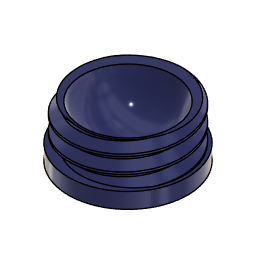
joint attachments v8 (Autodesk Fusion 360 archive; units mm, degrees)
design "thread"
Autodesk Fusion 360 part; units mm, degrees
sketch "Ball" plane through (0, 0, 0) normal (1, 0, 0) x (0, 1, 0)
  circle A0 centre (0, 0) radius 9 construction
  line L0 (0, 0) -> (0, 4.9749) construction
  line L1 (0, 4.9749) -> (-7.5, 4.9749) construction
  line L2 (-7.5, 4.9749) -> (-7.5, 0) construction
  line L3 (-7.5, 0) -> (-9, 0) construction
  line L4 (0, 0) -> (0, -2) construction
  line L5 (0, -2) -> (-8.775, -2) construction
  line L6 (0, -2) -> (0, -9) construction
  dimension "d58" = 18
  dimension "d109" = 2
  dimension "d110" = 1.5
  constraint coincident A0.centre L0.start
  constraint vertical L0
  constraint coincident A0 L1.end
  constraint perpendicular L0 L1
  constraint perpendicular L1 L2
  constraint coincident A0 L3.end
  constraint horizontal L3
  constraint coincident A0.centre L3
  constraint vertical L4
  constraint coincident A0 L5.end
  constraint perpendicular L4 L5
  constraint coincident A0 L6.end
  constraint perpendicular L5 L6
  measures "d58" diameter of A0
  measures "d109" distance of A0.centre L4.end
  measures "d110" distance of L2.end L3.end
sketch "Sketch1" plane through (0, 0, 0) normal (1, 0, 0) x (0, 1, 0) in component "Socket"
  circle A0 centre (0, 0) radius 9
  line L0 (0, -9) -> (-11.5, -9)
  line L1 (0, -12) -> (-11.5, -12)
  line L2 (-15, -2) -> (-15, -9)
  line L3 (-11.5, -12) -> (-11.5, -9)
  line L4 (0, -9) -> (0, -12)
  line L5 (0, -2) -> (-15, -2)
  line L6 (0, -2) -> (0, 0) construction
  line L7 (0, -2) -> (-8.775, -2) construction
  line L8 (0, -9) -> (-15, -9)
  dimension "d69" = 3
  dimension "d72" = 15
  dimension "d107" = 11.5
  constraint coincident L0 L2.end
  constraint horizontal L0
  constraint vertical L3
  constraint horizontal L1
  constraint coincident L1 L4.end
  constraint perpendicular L1 L4
  constraint coincident L1.start L4
  constraint vertical L2
  constraint horizontal L5
  constraint coincident L2.start L5.end
  constraint coincident A0.centre L6.end
  constraint vertical L6
  constraint coincident L4 A0.centre
  constraint coincident L0.start L4.start
  constraint coincident L5 L7.end
  constraint coincident A0 L0.start
  measures "d69" distance of L0.end L1.end
  measures "d72" distance of L5.start L2.start
  measures "d107" distance of L1.start L1.end
revolve "Revolve1" add sketch "Sketch1" angle 360 about axis through (0, 0, -2) along (0, 0, 1) contours A0 L0 L2 L5 L8 | L0 L1 L3 L4 L8 in component "Socket"
thread "Thread1" "ISO Metric profile 22.0 M22x3 6g" major diameter 21.7645 minor diameter 18.3374 pitch 3 angle 60 modelled right hand crest width 0.4298 on face at (-0.7477, -14.9814, -4.3333) crest through (0, -10.8823, -9.75) in component "Socket"
sketch "Angle Analysis" plane through (0, 0, 0) normal (1, 0, 0) x (0, 1, 0)
  line L0 (0, 0) -> (-4.0563, 6.5197)
  line L1 (0, 0) -> (0, 6.5197)
  dimension "MaxAngle" = 31.889
  constraint coincident L0.start L1.start
  constraint vertical L1
  constraint horizontal L0.end L1.end
  measures "MaxAngle" angle of L0 L1
component "Socket" placed x (1, 0, 0) y (0, 1, 0) z (0, 0, 1) at (0, 0, 0)
equation "d58 = BallDiameter"
equation "d69 = SocketFootThickness"
equation "d72 = BallDiameter / 2 + NutWallThickness"
equation "BallDiameter = 18 mm"
equation "BallClearance = 0.1 mm"
equation "NutWallThickness = 6 mm" comment "The thread size should be set to between BallDiameter and (BallDiameter+NutWallThickness)"
equation "BallFootToNutClearance = 1 mm" comment "How much smaller the foot of the ball is than the hole through the nut"
equation "BallFootThickness = 2 mm"
equation "SocketFootThickness = 3 mm"
equation "d107 = SocketFootWidth / 2"
equation "SocketFootWidth = 23 mm"
equation "d110 = BallToNutOverlap"
equation "KnurlWidth = 1.2 mm"
equation "BallToNutOverlap = 1.5 mm" comment "Smaller will increase the maximum angle but make the ball easier to pull through the nut"
equation "NutFilletRadius = 2 mm"
named bodies: "Socket"
